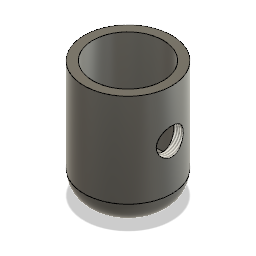
export1 (Autodesk Fusion 360 archive; units mm, degrees)
design "06_planter_container"
Autodesk Fusion 360 part; units mm, degrees
sketch "Sketch2" plane through (0, 0, 0) normal (0, 1, 0) x (1, 0, 0)
  circle A0 centre (0, 0) radius 75
  dimension "d1" = 150
  constraint coincident A0.centre origin
  measures "d1" diameter of A0
extrude "Extrude1" add sketch "Sketch2" along normal blind 200
fillet "Fillet1" radius 40 1 edges at (-69.9246, 0, 27.1212)
hole "Hole1" at (0, 200, 0) direction (0, -1, 0) diameter 120 depth 165 tip angle 118
hole "Hole2" at (75, 117.8728, 0) direction (-1, 0, 0) diameter 45.97 depth 50 tip angle 118
thread "Thread1" "ISO Metric profile 50.0 M50x4 6H"

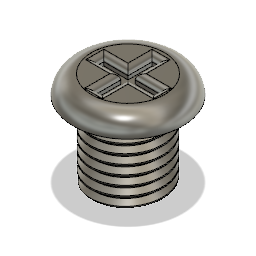
design "06_planter_screw"
Autodesk Fusion 360 part; units mm, degrees
sketch "Sketch2" plane through (0, 0, 0) normal (0, 0, 1) x (1, 0, 0)
  line L0 (0, 0) -> (10, 0)
  line L1 (10, 0) -> (10, 20)
  line L2 (10, 20) -> (15, 20)
  line L3 (15, 20) -> (15, 25)
  line L4 (15, 25) -> (0, 25)
  line L5 (0, 25) -> (0, 0)
  constraint coincident L0.start L5.end
  constraint horizontal L0
  constraint perpendicular L0 L1
  constraint perpendicular L1 L2
  constraint perpendicular L2 L3
  constraint perpendicular L3 L4
  constraint perpendicular L0 L5
revolve "Revolve1" add sketch "Sketch2" angle 360 about axis through (0, 25, 0) along (0, -1, 0)
sketch "Sketch3" plane through (0, 25, 0) normal (0, 1, 0) x (-1, 0, 0)
  circle A0 centre (0, 0) radius 15
  line L0 (1, -1) -> (1, -7.5984)
  line L1 (1, -7.5984) -> (-1, -7.5984)
  line L2 (-1, -7.5984) -> (-1, -1)
  line L3 (-1, -1) -> (-8, -1)
  line L4 (-8, -1) -> (-8, 1)
  line L5 (-8, 1) -> (-1, 1)
  line L6 (-1, 1) -> (-1, 8)
  line L7 (-1, 8) -> (1, 8)
  line L8 (1, 8) -> (1, 1)
  line L9 (1, 1) -> (7.6346, 1)
  line L10 (7.6346, 1) -> (7.6346, -1)
  line L11 (7.6346, -1) -> (1, -1)
  constraint perpendicular L0 L1
  constraint perpendicular L2 L3
  constraint perpendicular L3 L4
  constraint perpendicular L6 L7
  constraint perpendicular L9 L10
  constraint perpendicular L0 L11
extrude "Extrude2" cut sketch "Sketch3" against normal blind 2.5 contours L0 L1 L2 L3 L4 L5 L6 L7 L8 L9 L10 L11
fillet "Fillet1" radius 1.5 12 edges at (4.5, 25, 1) (8, 25, 0) (4.5, 25, -1) (1, 25, 4.5) (0, 25, 8) (-1, 25, 4.5) (-4.3173, 25, 1) (1, 25, -4.2992) (0, 25, -7.5984) (-1, 25, -4.2992) (-4.3173, 25, -1) (-7.6346, 25, 0)
fillet "Fillet2" radius 5 1 edges at (-13.9849, 25, -5.4242)
thread "Thread1" "ISO Metric profile 20.0 M20x2.5 6g" major diameter 19.7905 minor diameter 16.938 pitch 2.5 angle 60 modelled right hand crest width 0.36 on face at (9.9503, 13.3333, -0.9957) crest through (9.8953, 20.625, 0)
scale "Scale1" factor 1.5 about (-4.9183, 20, -6.8945) bodies 1
